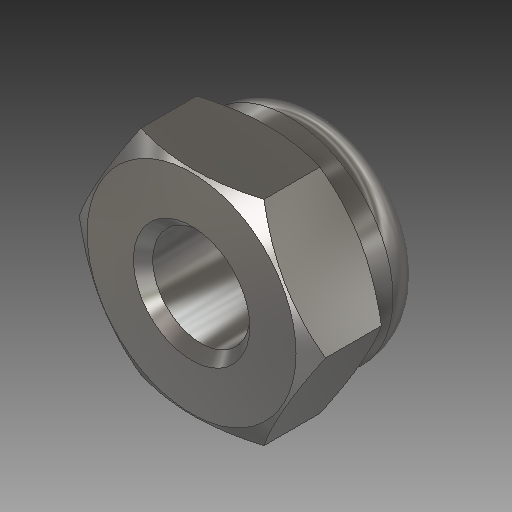
# Autodesk Inventor part: paris_nut
Saved by Autodesk Inventor 2019.3 (Build 233278000, 278)
## iProperties
Created: 2017-04-02
Part Number: paris_nut
Material: Типовые
Document SubType Name: Modeling
Designer: Nikita
Density: 1 g/cm^3
Appearance: Сталь — полированная
Mass: 0.518535 g
Surface Area: 4.84571 cm^2
Volume: 0.518535 cm^3
Author: Nikita
Autodesk Inventor part; units mm, degrees
ref_plane "YZ Plane" through (0, 0, 0) normal (1, 0, 0) x (0, 1, 0)
ref_plane "XZ Plane" through (0, 0, 0) normal (0, 1, 0) x (-1, 0, 0)
ref_plane "XY Plane" through (0, 0, 0) normal (0, 0, 1) x (1, 0, 0)
sketch "Эскиз1" plane through (0, 0, 0) normal (0, 0, 1) x (1, 0, 0)
  circle A0 centre (0, 0) radius 2.5
  line L0 (6.3509, 0) -> (3.1754, -5.5)
  line L1 (3.1754, -5.5) -> (-3.1754, -5.5)
  line L2 (-3.1754, -5.5) -> (-6.3509, 0)
  line L3 (-6.3509, 0) -> (-3.1754, 5.5)
  line L4 (-3.1754, 5.5) -> (3.1754, 5.5)
  line L5 (3.1754, 5.5) -> (6.3509, 0)
  dimension "d0" = 5
  dimension "d21" = 3
  constraints: 12 end point, 2 coincident, 1 centre point, 1 horizontal, 13 other
  measures "d0" diameter of A0
  measures "d21" distance edge to line of A0 L1
extrude "Выдавливание1" add sketch "Эскиз1" along normal blind 4
sketch "Эскиз2" plane through (0, 0, 0) normal (0, 1, 0) x (-1, 0, 0)
  line L0 (0, 0) -> (0, 12.9838)
  line L1 (-3.1754, 0) -> (-6.3509, 0) construction
  line L2 (-6.3509, 0) -> (-6.3509, 4) construction
  line L3 (-6.3509, 4) -> (-3.1754, 4) construction
  line L4 (-1.9952, -1.9581) -> (-8.8509, 2)
  line L5 (-8.8509, 2) -> (-1.9952, 5.9581)
  line L6 (-1.9952, 5.9581) -> (-9.8509, 5.9581)
  line L7 (-9.8509, 5.9581) -> (-9.8509, -1.9581)
  line L8 (-9.8509, -1.9581) -> (-1.9952, -1.9581)
  line L9 (-6.3509, 2) -> (-29.2681, 2) construction
  point P0 (-9.8509, 2)
  dimension "d4" = 60
  dimension "d5" = 1
  dimension "d6" = 3.5
  constraints: 14 end point, 2 horizontal, 2 midpoint, 2 perpendicular, 2 point on line, 1 vertical, 1 other
  measures "d4" angle of L5 L4
  measures "d5" distance from line of L7 L4.end
  measures "d6" distance between parallel lines of L2 L7
revolve "Вращение1" cut sketch "Эскиз2" angle 360 about axis through (0, 0, 0) along (0, 0, 1)
sketch "Эскиз3" plane through (0, 0, 0) normal (0, 0, -1) x (-1, 0, 0)
  circle A0 centre (0, 0) radius 2.5 projected
  circle A1 centre (0, 0) radius 5.3868 projected
  circle A2 centre (0, 0) radius 5.3868
  constraints: 1 centre point, 1 coincident, 1 concentric
extrude "Выдавливание2" add sketch "Эскиз3" along normal blind 3
fillet "Сопряжение1" radius 2 1 edges at (5.3868, 0, -3)
chamfer "Фаска2" distance 0.5 angle 45 1 edges at (-2.5, 0, 4)
sketch "Sketch5" plane through (0, 0, -3) normal (0, 0, -1) x (-1, 0, 0)
  circle A0 centre (0, 0) radius 2.5 projected
  circle A1 centre (0, 0) radius 3.3868 projected
extrude "Extrusion4" cut sketch "Sketch5" against normal blind 0.2
fillet "Fillet3" radius 0.2 1 edges at (3.3868, 0, -3)
